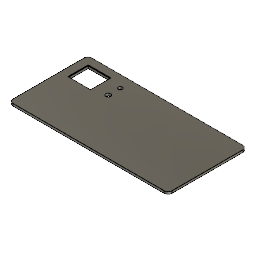
kkClave_Power_Panel v7 (Autodesk Fusion 360 design; units mm, degrees)
Autodesk Fusion 360 part; units mm, degrees
sketch "Sketch1" plane through (0, 0, 0) normal (0, 0, 1) x (1, 0, 0)
  line L0 (4.6495, 21.5388) -> (192.9573, 21.5388)
  line L1 (197.9573, 26.5388) -> (197.9573, 115.0177)
  line L2 (192.9573, 120.0177) -> (4.6495, 120.0177)
  line L3 (-0.3505, 115.0177) -> (-0.3505, 26.5388)
  line L4 (10, 110) -> (38, 110)
  line L5 (38, 110) -> (38, 85)
  line L6 (38, 85) -> (10, 85)
  line L7 (10, 85) -> (10, 110)
  circle A0 centre (55, 105) radius 2.5
  circle A1 centre (55, 90) radius 3.0001
  circle A2 centre (100, 105) radius 2.5
  circle A3 centre (100, 49) radius 2.5
  circle A4 centre (155, 105) radius 2.5
  circle A5 centre (155, 49) radius 2.5
  arc A6 (4.6495, 120.0177) -> (-0.3505, 115.0177) centre (4.6495, 115.0177) ccw
  arc A7 (197.9573, 115.0177) -> (192.9573, 120.0177) centre (192.9573, 115.0177) ccw
  arc A8 (192.9573, 21.5388) -> (197.9573, 26.5388) centre (192.9573, 26.5388) ccw
  arc A9 (-0.3505, 26.5388) -> (4.6495, 21.5388) centre (4.6495, 26.5388) ccw
  line L8 (4.6495, 115.0177) -> (192.9573, 115.0177)
  line L9 (192.9573, 115.0177) -> (192.9573, 26.5388)
  line L10 (192.9573, 26.5388) -> (4.6495, 26.5388)
  line L11 (4.6495, 26.5388) -> (4.6495, 115.0177)
  line L12 (8, 112) -> (189.9275, 112)
  line L13 (189.9275, 112) -> (189.9275, 29.9593)
  line L14 (189.9275, 29.9593) -> (8, 29.9593)
  line L15 (8, 29.9593) -> (8, 112)
  circle A10 centre (20, 40) radius 2
  circle A11 centre (20, 40) radius 3
  circle A12 centre (20, 75) radius 2
  circle A13 centre (20, 75) radius 3
  circle A14 centre (55, 40) radius 2
  circle A15 centre (55, 40) radius 3
  circle A16 centre (55, 75) radius 2
  circle A17 centre (55, 75) radius 3
  dimension "d1" = 5
  dimension "d2" = 6.0002
  dimension "d3" = 5
  dimension "d4" = 5
  dimension "d5" = 5
  dimension "d6" = 5
  dimension "d7" = 5
  constraint horizontal L0
  constraint vertical L1
  constraint horizontal L2
  constraint vertical L3
  constraint horizontal L4
  constraint vertical L5
  constraint horizontal L6
  constraint vertical L7
  constraint tangent L2 A6
  constraint tangent L3 A6
  constraint tangent L1 A7
  constraint tangent L2 A7
  constraint equal A6 A7
  constraint tangent L0 A8
  constraint tangent L1 A8
  constraint equal A6 A8
  constraint tangent L0 A9
  constraint tangent L3 A9
  constraint equal A6 A9
  constraint horizontal L8
  constraint vertical L9
  constraint vertical L11
  constraint coincident A8.centre L9.end
  constraint coincident A6.centre L8.start
  constraint horizontal L12
  constraint vertical L13
  constraint vertical L15
  constraint concentric A10 A11
  constraint concentric A12 A13
  constraint concentric A14 A15
  constraint concentric A16 A17
  measures "d1" diameter of A0
  measures "d2" diameter of A1
  measures "d3" diameter of A2
  measures "d4" diameter of A3
  measures "d5" diameter of A4
  measures "d6" diameter of A5
  measures "d7" radius of A6
extrude "Extrude8" add sketch "Sketch1" against normal blind 3 contours L0 L1 L2 L3 A6 A7 A8 A9 | L12 L13 L14 L15 makes body 1 at (67.4187, 23.2054, 0) makes body 2 at (118.9226, 85.7441, 0)
extrude "Extrude9" add sketch "Sketch1" against normal blind 6 contours L8 L9 L10 L11 bodies 1 2
extrude "Extrude10" add sketch "Sketch1" against normal blind 5 contours A11 | A13 | A15 | A17 bodies 1
extrude "Extrude11" add sketch "Sketch1" against normal blind 8 contours A10 | A12 | A14 | A16 bodies 1
extrude "Extrude12" add sketch "Sketch1" against normal blind 8 contours A2 | A3 | A4 | A5 bodies 1
chamfer "Chamfer4" distance 2 angle 45 1 edges at (10, 97.5, -3) on bodies 1
chamfer "Chamfer5" distance 2 angle 45 1 edges at (23, 110, -3) on bodies 1
chamfer "Chamfer6" distance 2 angle 45 1 edges at (38, 98.5, -3) on bodies 1
chamfer "Chamfer7" distance 2 angle 45 1 edges at (24, 85, -3) on bodies 1
